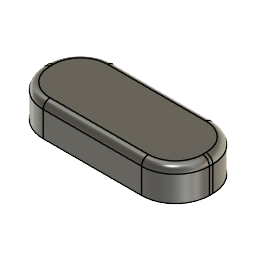
keycapX2 (Autodesk Fusion 360 design; units mm, degrees)
Autodesk Fusion 360 part; units mm, degrees
sketch "Sketch1" plane through (0, 0, 0) normal (0, 0, 1) x (1, 0, 0)
  line L0 (-0.6, 1) -> (-0.6, 2.15)
  line L1 (-0.6, 2.15) -> (0.6, 2.15)
  line L2 (0.6, 2.15) -> (0.6, 1)
  line L3 (0.9, 0.7) -> (2.15, 0.7)
  line L4 (2.15, 0.7) -> (2.15, -0.7)
  line L5 (2.15, -0.7) -> (0.9, -0.7)
  line L6 (0.6, -1) -> (0.6, -2.15)
  line L7 (0.6, -2.15) -> (-0.6, -2.15)
  line L8 (-0.6, -2.15) -> (-0.6, -1)
  line L9 (-0.9, -0.7) -> (-2.15, -0.7)
  line L10 (-2.15, -0.7) -> (-2.15, 0.7)
  line L11 (-2.15, 0.7) -> (-0.9, 0.7)
  arc A0 (-0.9, 0.7) -> (-0.6, 1) centre (-0.9, 1) ccw
  arc A1 (0.6, 1) -> (0.9, 0.7) centre (0.9, 1) ccw
  arc A2 (-0.6, -1) -> (-0.9, -0.7) centre (-0.9, -1) ccw
  arc A3 (0.9, -0.7) -> (0.6, -1) centre (0.9, -1) ccw
  circle A4 centre (0, 0) radius 3
  line L12 (28.9, 0.7) -> (30.15, 0.7)
  line L13 (27.4, 2.15) -> (28.6, 2.15)
  line L14 (28.6, -2.15) -> (27.4, -2.15)
  line L15 (30.15, 0.7) -> (30.15, -0.7)
  line L16 (25.85, -0.7) -> (25.85, 0.7)
  arc A5 (28.9, -0.7) -> (28.6, -1) centre (28.9, -1) ccw
  arc A6 (27.1, 0.7) -> (27.4, 1) centre (27.1, 1) ccw
  line L17 (28.6, 2.15) -> (28.6, 1)
  line L18 (27.4, -2.15) -> (27.4, -1)
  line L19 (30.15, -0.7) -> (28.9, -0.7)
  arc A7 (27.4, -1) -> (27.1, -0.7) centre (27.1, -1) ccw
  arc A8 (28.6, 1) -> (28.9, 0.7) centre (28.9, 1) ccw
  line L20 (27.4, 1) -> (27.4, 2.15)
  line L21 (27.1, -0.7) -> (25.85, -0.7)
  circle A9 centre (28, 0) radius 3
  line L22 (28.6, -1) -> (28.6, -2.15)
  line L23 (25.85, 0.7) -> (27.1, 0.7)
  point P0 (0.6, 0.7)
  point P1 (28.6, 0.7)
  point P2 (28, 0)
  dimension "d2" = 4.3
  dimension "d3" = 4.3
  dimension "d4" = 2.15
  dimension "d5" = 2.15
  dimension "d6" = 1.2
  dimension "d7" = 1.4
  dimension "d8" = 0.7
  dimension "d9" = 0.6
  dimension "d10" = 0.3
  dimension "d11" = 6
  dimension "d36" = 4.3
  dimension "d37" = 4.3
  dimension "d38" = 2.15
  dimension "d39" = 2.15
  dimension "d40" = 1.2
  dimension "d41" = 1.4
  dimension "d42" = 0.7
  dimension "d43" = 0.6
  dimension "d44" = 0.3
  dimension "d45" = 6
  dimension "d46" = 28
  constraint vertical L0
  constraint perpendicular L0 L1
  constraint perpendicular L1 L2
  constraint perpendicular L2 L3
  constraint perpendicular L3 L4
  constraint perpendicular L4 L5
  constraint perpendicular L3 L6
  constraint perpendicular L6 L7
  constraint perpendicular L7 L8
  constraint perpendicular L8 L9
  constraint perpendicular L7 L10
  constraint perpendicular L0 L11
  constraint tangent L0 A0
  constraint tangent L11 A0
  constraint coincident P0 L2
  constraint coincident P0 L3
  constraint tangent L2 A1
  constraint tangent L3 A1
  constraint equal A0 A1
  constraint tangent L8 A2
  constraint tangent L9 A2
  constraint equal A0 A2
  constraint tangent L5 A3
  constraint tangent L6 A3
  constraint equal A0 A3
  constraint horizontal P0 L11.end
  constraint horizontal L9.start L5.end
  constraint vertical L0.start L8.end
  constraint vertical P0 L6.start
  constraint coincident A4.centre origin
  constraint vertical L20
  constraint perpendicular L13 L20
  constraint perpendicular L13 L17
  constraint perpendicular L12 L17
  constraint perpendicular L12 L15
  constraint perpendicular L15 L19
  constraint perpendicular L12 L22
  constraint perpendicular L14 L22
  constraint perpendicular L14 L18
  constraint perpendicular L18 L21
  constraint perpendicular L14 L16
  constraint perpendicular L20 L23
  constraint tangent A6 L20
  constraint tangent A6 L23
  constraint coincident P1 L17
  constraint coincident P1 L12
  constraint tangent L17 A8
  constraint tangent L12 A8
  constraint equal A6 A8
  constraint tangent L18 A7
  constraint tangent A7 L21
  constraint equal A6 A7
  constraint tangent A5 L19
  constraint tangent A5 L22
  constraint equal A5 A6
  constraint horizontal P1 A6.start
  constraint horizontal A7.end A5.start
  constraint vertical A6.end L18.end
  constraint vertical P1 A5.end
  constraint coincident P2 A9.centre
  constraint horizontal A4.centre P2
  measures "d2" distance of L4 L10
  measures "d3" distance of L1 L7
  measures "d4" distance of A4.centre L4
  measures "d5" distance of A4.centre L7
  measures "d6" distance of L0.end L1.end
  measures "d7" distance of L3.end L4.end
  measures "d8" vertical distance of A4.centre P0
  measures "d9" horizontal distance of A4.centre P0
  measures "d10" radius of A0
  measures "d11" diameter of A4
  measures "d36" distance of L15 L16
  measures "d37" distance of L13 L14
  measures "d38" distance of P2 L15
  measures "d39" distance of P2 L14
  measures "d40" distance of L13.start L13.end
  measures "d41" distance of L12.end L15.end
  measures "d42" vertical distance of P1 P2
  measures "d43" horizontal distance of P1 P2
  measures "d44" radius of A6
  measures "d45" diameter of A9
  measures "d46" distance of A4.centre P2
extrude "Extrude1" add sketch "Sketch1" along normal blind 7 makes body 1 at (2.9851, -0.2987, 4.6667) makes body 2 at (30.9851, -0.2987, 4.6667)
sketch "Sketch2" plane through (0, 0, 7) normal (0, 0, 1) x (-1, 0, 0)
  line L0 (-2.15, 0.7) -> (-0.9, 0.7)
  arc A0 (-0.9, 0.7) -> (-0.6, 1) centre (-0.9, 1) ccw
  line L1 (-0.6, 1) -> (-0.6, 2.15)
  line L2 (-0.6, 2.15) -> (0.6, 2.15)
  line L3 (0.6, 2.15) -> (0.6, 1)
  arc A1 (0.6, 1) -> (0.9, 0.7) centre (0.9, 1) ccw
  line L4 (0.9, 0.7) -> (2.15, 0.7)
  line L5 (2.15, 0.7) -> (2.15, -0.7)
  line L6 (2.15, -0.7) -> (0.9, -0.7)
  arc A2 (0.9, -0.7) -> (0.6, -1) centre (0.9, -1) ccw
  line L7 (0.6, -1) -> (0.6, -2.15)
  line L8 (0.6, -2.15) -> (-0.6, -2.15)
  line L9 (-0.6, -2.15) -> (-0.6, -1)
  arc A3 (-0.6, -1) -> (-0.9, -0.7) centre (-0.9, -1) ccw
  line L10 (-0.9, -0.7) -> (-2.15, -0.7)
  line L11 (-2.15, -0.7) -> (-2.15, 0.7)
  circle A4 centre (0, 0) radius 3
  line L12 (10.5, 10.5) -> (-38.5, 10.5)
  line L13 (-38.5, 10.5) -> (-38.5, -10.5)
  line L14 (-38.5, -10.5) -> (10.5, -10.5)
  line L15 (10.5, -10.5) -> (10.5, 10.5)
  dimension "d15" = 21
  dimension "d16" = 10.5
  dimension "d17" = 10.5
  dimension "d47" = 38.5
  constraint horizontal L12
  constraint vertical L13
  constraint horizontal L14
  constraint vertical L15
  measures "d15" distance of L12.start L14.end
  measures "d16" horizontal distance of A4.centre L12.start
  measures "d17" vertical distance of A4.centre L12.start
  measures "d47" distance of A4.centre L13
extrude "Extrude2" add sketch "Sketch2" along normal blind 2 contours L0 A0 L1 L2 L3 A1 L4 L5 L6 A2 L7 L8 L9 A3 L10 L11 | A4 | L12 L13 L14 L15 bodies 1 2
sketch "Sketch3" plane through (0, 0, 7) normal (0, 0, -1) x (1, 0, 0)
  line L0 (-10.5, 10.5) -> (-10.5, -10.5)
  line L1 (-10.5, -10.5) -> (38.5, -10.5)
  line L2 (38.5, -10.5) -> (38.5, 10.5)
  line L3 (38.5, 10.5) -> (-10.5, 10.5)
  circle A0 centre (0, 0) radius 3
  line L4 (38.5, -10.5) -> (-10.5, -10.5)
  line L5 (-10.5, -10.5) -> (-10.5, 10.5)
  line L6 (-10.5, 10.5) -> (38.5, 10.5)
  line L7 (38.5, 10.5) -> (38.5, -10.5)
  line L8 (-8.9, 8.9) -> (36.9, 8.9)
  line L9 (36.9, 8.9) -> (36.9, -8.9)
  line L10 (36.9, -8.9) -> (-8.9, -8.9)
  line L11 (-8.9, -8.9) -> (-8.9, 8.9)
  circle A1 centre (28, 0) radius 3
  dimension "d20" = 1.6
  dimension "d21" = 1.6
  dimension "d22" = 1.6
  dimension "d23" = 1.6
  constraint horizontal L4
  constraint vertical L5
  constraint horizontal L6
  constraint vertical L7
  constraint coincident L0.start L3.end
  constraint coincident L1.end L2.start
  constraint horizontal L8
  constraint vertical L9
  constraint horizontal L10
  constraint vertical L11
  measures "d20" vertical distance of L1.end L9.end
  measures "d21" horizontal distance of L1.end L9.end
  measures "d22" horizontal distance of L0.end L10.end
  measures "d23" vertical distance of L0.start L8.start
extrude "Extrude3" add sketch "Sketch3" along normal blind 7.5 contours L0 L1 L2 L3 L4 L5 L6 L7 bodies 1
fillet "Fillet1" radius 3 1 faces at (18.3013, 6.8642, 7) on bodies 1
fillet "Fillet1" radius 8.4 4 edges at (-8.9, -8.9, 3.25) (-8.9, 8.9, 3.25) (36.9, 8.9, 3.25) (36.9, -8.9, 3.25) on bodies 1
fillet "Fillet1" radius 10 4 edges at (-10.5, -10.5, 4.25) (-10.5, 10.5, 4.25) (38.5, -10.5, 4.25) (38.5, 10.5, 4.25) on bodies 1
fillet "Fillet1" radius 2 1 faces at (22.1667, 3.5, 9) on bodies 1
extrude "Extrude4" add 2 faces at (-0.2345, 0.2578, 7) (27.7655, -0.2578, 7) along direction (0, 0, -1) blind 3.3 on bodies 1 bodies 1
equation "d8 = ( 1.4 / 2 ) * 1 mm"
equation "d9 = ( 1.2 / 2 ) * 1 mm"
equation "d16 = ( 21 / 2 ) * 1 mm"
equation "d17 = ( 21 / 2 ) * 1 mm"
equation "d34 = 7 mm - 3.7 mm"
equation "d42 = ( 1.4 / 2 ) * 1 mm"
equation "d43 = ( 1.2 / 2 ) * 1 mm"
equation "d47 = 28 mm + ( 21 / 2 ) * 1 mm"
